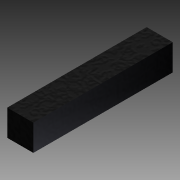
# Autodesk Inventor part: Ad-hoc 3!16 axle key
Saved by Autodesk Inventor 2011 SP1 (Build 150282100, 282)
## iProperties
Created: 2011-01-12
Part Number: Ad-hoc 3!16 axle key
Document SubType Name: Modeling
Designer: Christopher
Density: 1 g/cm^3
Author: Christopher
Autodesk Inventor part; units mm, degrees
ref_plane "YZ Plane" through (0, 0, 0) normal (1, 0, 0) x (0, 1, 0)
ref_plane "XZ Plane" through (0, 0, 0) normal (0, 1, 0) x (-1, 0, 0)
ref_plane "XY Plane" through (0, 0, 0) normal (0, 0, 1) x (1, 0, 0)
sketch "Sketch1" plane through (0, 0, 0) normal (0, 0, 1) x (1, 0, 0)
  line L0 (-15.7287, 11.544) -> (-10.9662, 11.544)
  line L1 (-10.9662, 11.544) -> (-10.9662, 6.7815)
  line L2 (-10.9662, 6.7815) -> (-15.7287, 6.7815)
  line L3 (-15.7287, 6.7815) -> (-15.7287, 11.544)
  point P0 (0, 0)
  dimension "d0" = 4.7625
  dimension "d1" = 4.7625
  constraints: 8 end point, 2 parallel, 1 horizontal, 1 perpendicular
  measures "d0" distance of L0.start L0.end
  measures "d1" distance of L2.end L0.start
extrude "Extrusion1" add sketch "Sketch1" against normal blind 25.4
body "Solid1"
